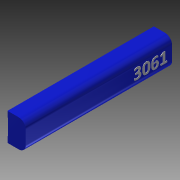
# Autodesk Inventor part: Bumper Cover Part1 (26x28 robot)
Saved by Autodesk Inventor 2014 SP1 (Build 180222100, 222)
## iProperties
Created: 2013-01-06
Part Number: Bumper Cover Part1 (26x28 robot)
Material: Generic
Document SubType Name: Modeling
Designer: Moses
Density: 1 g/cm^3
Mass: 387.925 g
Surface Area: 4847.49 cm^2
Volume: 387.925 cm^3
Appearance: Blue - Wall Paint - Glossy
Author: Moses
Autodesk Inventor part; units mm, degrees
ref_plane "YZ Plane" through (0, 0, 0) normal (1, 0, 0) x (0, 1, 0)
ref_plane "XZ Plane" through (0, 0, 0) normal (0, 1, 0) x (-1, 0, 0)
ref_plane "XY Plane" through (0, 0, 0) normal (0, 0, 1) x (1, 0, 0)
sketch "Sketch1" plane through (0, 0, 0) normal (0, 0, 1) x (1, 0, 0)
  circle A0 centre (38.1, -31.75) radius 31.75 construction
  circle A1 centre (38.1, 31.75) radius 31.75 construction
  line L0 (6.35, 63.5) -> (38.1, 63.5) construction
  line L1 (69.85, 31.75) -> (69.85, -31.75) construction
  line L2 (6.35, -63.5) -> (38.1, -63.5) construction
  line L3 (38.1, 65.0875) -> (-14.2875, 65.0875)
  line L4 (-14.2875, -65.0875) -> (38.1, -65.0875)
  arc A2 (38.1, -65.0875) -> (71.4375, -31.75) centre (38.1, -31.75) ccw
  arc A3 (71.4375, 31.75) -> (38.1, 65.0875) centre (38.1, 31.75) ccw
  line L5 (71.4375, 31.75) -> (71.4375, -31.75)
  line L6 (38.1, 65.0875) -> (38.1, 63.5) construction
  arc A4 (69.85, 31.75) -> (38.1, 63.5) centre (38.1, 31.75) ccw
  arc A5 (38.1, -63.5) -> (69.85, -31.75) centre (38.1, -31.75) ccw
  line L7 (69.85, 31.75) -> (69.85, -31.75)
  line L8 (-12.7, 63.5) -> (-12.7, 38.1)
  line L9 (-12.7, 38.1) -> (-14.2875, 38.1)
  line L10 (-14.2875, 38.1) -> (-14.2875, 65.0875)
  line L11 (-14.2875, -65.0875) -> (-14.2875, -38.1)
  line L12 (-14.2875, -38.1) -> (-12.7, -38.1)
  line L13 (-12.7, -63.5) -> (-12.7, -38.1)
  line L14 (-12.7, 38.1) -> (-12.7, -38.1)
  line L15 (6.35, -63.5) -> (6.35, 63.5) construction
  line L16 (6.35, 63.5) -> (-12.7, 63.5) construction
  line L17 (-12.7, 63.5) -> (-12.7, -63.5) construction
  line L18 (-12.7, -63.5) -> (6.35, -63.5) construction
  line L19 (-12.7, 63.5) -> (38.1, 63.5)
  line L20 (-12.7, -63.5) -> (38.1, -63.5)
  point P0 (0, 0)
  point P1 (38.1, 64.2937)
  dimension "d3" = 25.4
  dimension "d7" = 25.4
  dimension "d9" = 1.5875
  dimension "d45" = 1.5875
  dimension "d46" = 1.5875
  constraints: 34 end point, 14 tangent, 12 point on circle, 4 centre point, 4 perpendicular, 3 collinear, 3 parallel, 2 coincident, 2 point on line, 1 concentric, 1 midpoint, 1 vertical
  measures "d3" distance of L8.start L8.end
  measures "d7" distance of L13.start L12.end
  measures "d9" distance of L3.start L0.end
  measures "d45" distance of L11.end L12.end
  measures "d46" distance of L8.end L9.end
extrude "Extrusion1" add sketch "Sketch1" along normal blind 1.5875
extrude "Extrusion2" add sketch "Sketch1" against normal blind 682.625 contours A3 L5 A2 L4 L11 L12 L13 L20 A5 L7 A4 L19 L8 L9 L10 L3
sketch "Sketch2" plane through (0, 0, -682.625) normal (0, 0, -1) x (-1, 0, 0)
  arc A0 (-38.1, 63.5) -> (-69.85, 31.75) centre (-38.1, 31.75) ccw projected
  line L0 (-38.1, 63.5) -> (12.7, 63.5) projected
  line L1 (12.7, 63.5) -> (12.7, 38.1) projected
  line L2 (12.7, 38.1) -> (14.2875, 38.1) projected
  line L3 (14.2875, 38.1) -> (14.2875, 65.0875) projected
  line L4 (14.2875, 65.0875) -> (-38.1, 65.0875) projected
  arc A1 (-38.1, 65.0875) -> (-71.4375, 31.75) centre (-38.1, 31.75) ccw projected
  line L5 (-71.4375, 31.75) -> (-71.4375, -31.75) projected
  arc A2 (-71.4375, -31.75) -> (-38.1, -65.0875) centre (-38.1, -31.75) ccw projected
  line L6 (-38.1, -65.0875) -> (14.2875, -65.0875) projected
  line L7 (14.2875, -65.0875) -> (14.2875, -38.1) projected
  line L8 (14.2875, -38.1) -> (12.7, -38.1) projected
  line L9 (12.7, -38.1) -> (12.7, -63.5) projected
  line L10 (12.7, -63.5) -> (-38.1, -63.5) projected
  arc A3 (-69.85, -31.75) -> (-38.1, -63.5) centre (-38.1, -31.75) ccw projected
  line L11 (-69.85, -31.75) -> (-69.85, 31.75) projected
  line L12 (12.7, -63.5) -> (12.7, 63.5) projected
extrude "Extrusion3" add sketch "Sketch2" along normal blind 1.5875
sketch "Sketch3" plane through (71.4375, -31.75, 1.5875) normal (1, 0, 0) x (0, 0, -1)
  line L0 (508, 63.5) -> (660.4, 63.5) construction
  line L1 (660.4, 63.5) -> (660.4, 0) construction
  line L2 (660.4, 0) -> (508, 0) construction
  line L3 (508, 0) -> (508, 63.5) construction
  line L4 (685.8, 31.75) -> (0, 31.75) construction
  line L5 (685.8, 63.5) -> (685.8, 0) construction
  line L6 (0, 0) -> (0, 63.5) construction
  line L7 (685.8, 63.5) -> (0, 63.5) construction
  line L8 (685.8, 0) -> (0, 0) construction
  spline S0 degree 2 poles (540.2687, 21.2561) (540.2687, 17.4878) (537.3591, 11.6208) (532.2075, 7.614) (525.0049, 5.563) (520.7596, 5.563) knots 0 0 0 1 2 3 4 4 4
  spline S1 degree 2 poles (520.7596, 5.563) (518.1839, 5.563) (513.6524, 6.3262) (510.1703, 7.3755) (507.8808, 8.568) (507.213, 9.1881) (506.8314, 9.999) (506.5452, 11.0484) (506.4498, 12.6225) (506.4498, 13.7673) knots 0 0 0 1 2 3 4 5 6 7 8 8 8
  spline S2 degree 2 poles (506.4498, 13.7673) (506.4498, 15.6753) (507.0699, 17.1062) (507.69, 17.1062) knots 0 0 0 1 2 2 2
  spline S3 degree 2 poles (507.69, 17.1062) (508.0716, 17.1062) (510.0272, 16.0569) (512.9846, 14.8167) (516.9914, 13.7673) (519.5194, 13.7673) knots 0 0 0 1 2 3 4 4 4
  spline S4 degree 2 poles (519.5194, 13.7673) (521.6659, 13.7673) (524.9572, 14.769) (527.2468, 16.6293) (528.3915, 19.2527) (528.3915, 20.8268) knots 0 0 0 1 2 3 4 4 4
  spline S5 degree 2 poles (528.3915, 20.8268) (528.3915, 22.5917) (527.0083, 25.406) (524.3371, 27.4093) (520.2349, 28.5064) (517.4207, 28.5064) knots 0 0 0 1 2 3 4 4 4
  line L9 (517.4207, 28.5064) -> (513.0323, 28.5064)
  spline S6 degree 2 poles (513.0323, 28.5064) (512.5553, 28.5064) (511.8398, 28.7926) (511.3628, 29.6512) (511.172, 31.1776) (511.172, 32.3701) knots 0 0 0 1 2 3 4 4 4
  spline S7 degree 2 poles (511.172, 32.3701) (511.172, 33.5149) (511.3628, 34.9459) (511.7921, 35.7091) (512.4599, 36.043) (512.9369, 36.043) knots 0 0 0 1 2 3 4 4 4
  line L10 (512.9369, 36.043) -> (517.373, 36.043)
  spline S8 degree 2 poles (517.373, 36.043) (519.6625, 36.043) (523.1923, 37.0923) (525.5773, 39.048) (526.8175, 41.8146) (526.8175, 43.5318) knots 0 0 0 1 2 3 4 4 4
  spline S9 degree 2 poles (526.8175, 43.5318) (526.8175, 44.8197) (525.9589, 47.1092) (524.2894, 48.7787) (521.6182, 49.7804) (519.8056, 49.7804) knots 0 0 0 1 2 3 4 4 4
  spline S10 degree 2 poles (519.8056, 49.7804) (517.7546, 49.7804) (514.1771, 48.5879) (511.3151, 47.1092) (509.3117, 45.8691) (508.8347, 45.8691) knots 0 0 0 1 2 3 4 4 4
  spline S11 degree 2 poles (508.8347, 45.8691) (508.5485, 45.8691) (508.0716, 46.1553) (507.7377, 46.9185) (507.5946, 48.3971) (507.5946, 49.5896) knots 0 0 0 1 2 3 4 4 4
  spline S12 degree 2 poles (507.5946, 49.5896) (507.5946, 50.5436) (507.69, 51.8315) (507.9285, 52.6901) (508.2623, 53.3102) (509.0255, 54.0734) (511.4582, 55.5521) (515.1311, 56.9831) (519.9487, 57.937) (522.763, 57.937) knots 0 0 0 1 2 3 4 5 6 7 8 8 8
  spline S13 degree 2 poles (522.763, 57.937) (526.4359, 57.937) (532.1121, 56.2199) (535.9758, 52.9763) (537.9792, 48.254) (537.9792, 45.249) knots 0 0 0 1 2 3 4 4 4
  spline S14 degree 2 poles (537.9792, 45.249) (537.9792, 42.9594) (536.7867, 39.0003) (534.5448, 35.8522) (531.1104, 33.658) (528.9162, 33.1333) knots 0 0 0 1 2 3 4 4 4
  line L11 (528.9162, 33.1333) -> (528.9162, 32.9902)
  spline S15 degree 2 poles (528.9162, 32.9902) (531.5397, 32.704) (535.785, 30.6052) (538.6946, 27.5047) (540.2687, 23.5457) (540.2687, 21.2561) knots 0 0 0 1 2 3 4 4 4
  spline S16 degree 2 poles (582.0535, 31.9408) (582.0535, 25.883) (580.0978, 16.1046) (575.6618, 9.2358) (568.6023, 5.563) (563.4984, 5.563) knots 0 0 0 1 2 3 4 4 4
  spline S17 degree 2 poles (563.4984, 5.563) (558.2992, 5.563) (551.4781, 9.1404) (547.5191, 15.8184) (545.8973, 25.4537) (545.8973, 31.5592) knots 0 0 0 1 2 3 4 4 4
  spline S18 degree 2 poles (545.8973, 31.5592) (545.8973, 37.5693) (547.9007, 47.3954) (552.289, 54.2642) (559.3962, 57.937) (564.4524, 57.937) knots 0 0 0 1 2 3 4 4 4
  spline S19 degree 2 poles (564.4524, 57.937) (569.6516, 57.937) (576.5204, 54.3596) (580.4794, 47.6816) (582.0535, 38.0463) (582.0535, 31.9408) knots 0 0 0 1 2 3 4 4 4
  spline S20 degree 2 poles (571.7027, 31.4638) (571.7027, 35.0413) (571.3211, 40.5744) (570.5102, 44.6289) (569.27, 47.4431) (567.5529, 49.1126) (565.3587, 49.8281) (564.0231, 49.8281) knots 0 0 0 1 2 3 4 5 6 6 6
  spline S21 degree 2 poles (564.0231, 49.8281) (561.7335, 49.8281) (558.7285, 47.5862) (556.9636, 43.1502) (556.2481, 36.4723) (556.2481, 32.0839) knots 0 0 0 1 2 3 4 4 4
  spline S22 degree 2 poles (556.2481, 32.0839) (556.2481, 26.6462) (557.1067, 19.5866) (558.9669, 15.3891) (561.8289, 13.7196) (563.88, 13.7196) knots 0 0 0 1 2 3 4 4 4
  spline S23 degree 2 poles (563.88, 13.7196) (565.4064, 13.7196) (567.7437, 14.7213) (569.5085, 16.6769) (570.701, 19.6343) (571.4165, 23.5457) (571.7027, 28.4587) (571.7027, 31.4638) knots 0 0 0 1 2 3 4 5 6 6 6
  spline S24 degree 2 poles (622.3596, 23.3549) (622.3596, 19.5389) (620.0223, 13.0041) (615.4909, 8.2818) (608.813, 5.563) (604.4723, 5.563) knots 0 0 0 1 2 3 4 4 4
  spline S25 degree 2 poles (604.4723, 5.563) (600.9902, 5.563) (595.7433, 7.1847) (591.9273, 10.1898) (589.4946, 14.4828) (588.016, 19.8728) (587.4913, 26.2169) (587.4913, 29.7466) knots 0 0 0 1 2 3 4 5 6 6 6
  spline S26 degree 2 poles (587.4913, 29.7466) (587.4913, 32.704) (588.0637, 39.1911) (589.7808, 45.4398) (592.8336, 51.116) (597.6036, 55.409) (604.4723, 57.8893) (609.1469, 57.8893) knots 0 0 0 1 2 3 4 5 6 6 6
  spline S27 degree 2 poles (609.1469, 57.8893) (610.6255, 57.8893) (613.6783, 57.5554) (616.2541, 56.9831) (618.019, 56.2676) (618.6391, 55.7906) (618.9253, 55.1705) (619.1161, 54.4073) (619.2115, 53.3102) (619.2115, 52.547) knots 0 0 0 1 2 3 4 5 6 7 8 8 8
  spline S28 degree 2 poles (619.2115, 52.547) (619.2115, 51.3068) (619.1161, 49.685) (618.7822, 48.8264) (618.2098, 48.3971) (617.8282, 48.3971) knots 0 0 0 1 2 3 4 4 4
  spline S29 degree 2 poles (617.8282, 48.3971) (617.3512, 48.3971) (615.8725, 48.9218) (613.7737, 49.5419) (610.9117, 50.0189) (609.0515, 50.0189) knots 0 0 0 1 2 3 4 4 4
  spline S30 degree 2 poles (609.0515, 50.0189) (605.8556, 50.0189) (601.4672, 47.6816) (598.7484, 43.6749) (597.5082, 38.3802) (597.4605, 35.4229) knots 0 0 0 1 2 3 4 4 4
  spline S31 degree 2 poles (597.4605, 35.4229) (598.3191, 35.9476) (600.5609, 37.0446) (603.1844, 37.8078) (606.1895, 38.3325) (607.9544, 38.3325) knots 0 0 0 1 2 3 4 4 4
  spline S32 degree 2 poles (607.9544, 38.3325) (611.7703, 38.3325) (617.2558, 36.2338) (620.7378, 32.3224) (622.3596, 26.7416) (622.3596, 23.3549) knots 0 0 0 1 2 3 4 4 4
  spline S33 degree 2 poles (612.295, 22.4009) (612.295, 24.3566) (611.5795, 27.4093) (610.0054, 29.4604) (607.4297, 30.5098) (605.6171, 30.5098) knots 0 0 0 1 2 3 4 4 4
  spline S34 degree 2 poles (605.6171, 30.5098) (604.52, 30.5098) (602.3735, 30.1282) (600.3701, 29.4127) (598.4622, 28.4587) (597.6513, 27.8863) knots 0 0 0 1 2 3 4 4 4
  spline S35 degree 2 poles (597.6513, 27.8863) (597.6513, 23.7365) (598.6053, 18.1079) (600.4178, 14.8644) (603.2321, 13.4811) (605.0447, 13.4811) knots 0 0 0 1 2 3 4 4 4
  spline S36 degree 2 poles (605.0447, 13.4811) (606.8573, 13.4811) (609.5761, 14.8167) (611.341, 17.2493) (612.295, 20.4929) (612.295, 22.4009) knots 0 0 0 1 2 3 4 4 4
  spline S37 degree 2 poles (661.664, 10.3806) (661.664, 9.2835) (661.4255, 7.7571) (660.9962, 6.8508) (660.4715, 6.4693) (660.09, 6.4693) knots 0 0 0 1 2 3 4 4 4
  line L12 (660.09, 6.4693) -> (632.1857, 6.4693)
  spline S38 degree 2 poles (632.1857, 6.4693) (631.8518, 6.4693) (631.3271, 6.8508) (630.8978, 7.7571) (630.6593, 9.2835) (630.6593, 10.3806) knots 0 0 0 1 2 3 4 4 4
  spline S39 degree 2 poles (630.6593, 10.3806) (630.6593, 11.4777) (630.8501, 13.0041) (631.2794, 13.9581) (631.8518, 14.3874) (632.1857, 14.3874) knots 0 0 0 1 2 3 4 4 4
  line L13 (632.1857, 14.3874) -> (641.5825, 14.3874)
  line L14 (641.5825, 14.3874) -> (641.5825, 47.3477)
  line L15 (641.5825, 47.3477) -> (633.4259, 42.864)
  spline S40 degree 2 poles (633.4259, 42.864) (632.5673, 42.4347) (631.4225, 42.2439) (630.7547, 42.9117) (630.5162, 44.5335) (630.5162, 46.0122) knots 0 0 0 1 2 3 4 4 4
  spline S41 degree 2 poles (630.5162, 46.0122) (630.5162, 46.9662) (630.6116, 48.1586) (630.8978, 49.0172) (631.4702, 49.5896) (631.9472, 49.8758) knots 0 0 0 1 2 3 4 4 4
  line L16 (631.9472, 49.8758) -> (642.775, 56.8877)
  spline S42 degree 2 poles (642.775, 56.8877) (643.0135, 57.0785) (643.5859, 57.2692) (644.5399, 57.3646) (646.0663, 57.4123) (647.2588, 57.4123) knots 0 0 0 1 2 3 4 4 4
  spline S43 degree 2 poles (647.2588, 57.4123) (648.7375, 57.4123) (650.5977, 57.3169) (651.504, 57.0308) (651.8379, 56.5538) (651.8379, 56.2199) knots 0 0 0 1 2 3 4 4 4
  line L17 (651.8379, 56.2199) -> (651.8379, 14.3874)
  line L18 (651.8379, 14.3874) -> (660.09, 14.3874)
  spline S44 degree 2 poles (660.09, 14.3874) (660.4715, 14.3874) (661.0439, 13.9581) (661.4732, 13.0041) (661.664, 11.4777) (661.664, 10.3806) knots 0 0 0 1 2 3 4 4 4
  point P0 (660.4, 31.75)
  dimension "d0" = 1.5875
  dimension "d1" = 0
  dimension "d42" = 152.4
  dimension "d47" = 25.4
  dimension "d48" = 63.5
  constraints: 6 midpoint, 2 end point, 2 point on line, 2 other
  measures "d42" distance between parallel lines of L1 L3
  measures "d47" distance between parallel lines of L5 L1
  measures "d48" distance of L2.end L0.start
extrude "Extrusion5" add sketch "Sketch3" along normal blind 1.5875
body "Solid1"
